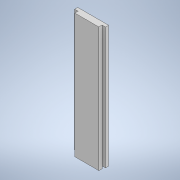
# Autodesk Inventor part: magea
Saved by Autodesk Inventor 2022 (Build 260153000, 153)
## iProperties
Created: 2021-11-19
Part Number: magea
Material: 일반
Document SubType Name: Modeling
Designer: ELEC-01
Density: 1 g/cm^3
Appearance: 기본값
Author: ELEC-01
Autodesk Inventor part; units mm, degrees
ref_plane "YZ Plane" through (0, 0, 0) normal (1, 0, 0) x (0, 1, 0)
ref_plane "XZ Plane" through (0, 0, 0) normal (0, 1, 0) x (-1, 0, 0)
ref_plane "XY Plane" through (0, 0, 0) normal (0, 0, 1) x (1, 0, 0)
sketch "스케치1" plane through (0, 0, 0) normal (0, 0, 1) x (1, 0, 0)
  line L0 (0, 0) -> (19, 0)
  line L1 (19, 0) -> (19, 75)
  line L2 (19, 75) -> (0, 75)
  line L3 (0, 75) -> (0, 0)
  dimension "d0" = 19
  dimension "d1" = 75
  constraints: 8 end point, 2 parallel, 1 horizontal, 1 perpendicular
  measures "d0" distance of L2.end L1.end
  measures "d1" distance of L2.end L0.start
extrude "돌출1" add sketch "스케치1" along normal blind 1.9
sketch "스케치2" plane through (0, 0, 1.9) normal (0, 0, 1) x (1, 0, 0)
  line L0 (2.1, 75) -> (16.9, 75)
  line L1 (16.9, 75) -> (16.9, -1.5)
  line L2 (16.9, -1.5) -> (2.1, -1.5)
  line L3 (2.1, -1.5) -> (2.1, 75)
  line L4 (19, 75) -> (0, 75) projected
  line L5 (0, 75) -> (0, 0) projected
  line L6 (19, 0) -> (19, 75) projected
  dimension "d4" = 0
  dimension "d5" = 2.1
  dimension "d6" = 2.1
  dimension "d7" = 76.5
  constraints: 8 end point, 2 parallel, 1 horizontal, 1 perpendicular
  measures "d4" distance between parallel lines of L4 L0
  measures "d5" distance between parallel lines of L5 L3
  measures "d6" distance between parallel lines of L6 L1
  measures "d7" distance between parallel lines of L0 L2
extrude "돌출2" add sketch "스케치2" along normal blind 2
